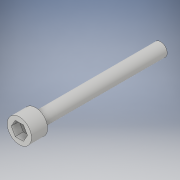
# Autodesk Inventor part: RobotArm Rivet2
Saved by Autodesk Inventor 2018 (Build 220112000, 112)
## iProperties
Created: 2018-01-20
Part Number: RobotArm Rivet2
Material: Generic
Document SubType Name: Modeling
Designer: lopez.xavier
Density: 1 g/cm^3
Appearance: Default
Author: lopez.xavier
Autodesk Inventor part; units mm, degrees
ref_plane "YZ Plane" through (0, 0, 0) normal (1, 0, 0) x (0, 1, 0)
ref_plane "XZ Plane" through (0, 0, 0) normal (0, 1, 0) x (-1, 0, 0)
ref_plane "XY Plane" through (0, 0, 0) normal (0, 0, 1) x (1, 0, 0)
sketch "Sketch1" plane through (0, 0, 0) normal (0, 0, 1) x (1, 0, 0)
  circle A0 centre (0, 0) radius 3.81
  dimension "d0" = 7.62
  constraints: 1 centre point, 1 coincident
  measures "d0" diameter of A0
extrude "Extrusion1" add sketch "Sketch1" along normal blind 5.08
sketch "Sketch2" plane through (0, 0, 5.08) normal (0, 0, 1) x (1, 0, 0)
  line L0 (1.2832, 2.2225) -> (2.5663, 0)
  line L1 (2.5663, 0) -> (1.2832, -2.2225)
  line L2 (1.2832, -2.2225) -> (-1.2832, -2.2225)
  line L3 (-1.2832, -2.2225) -> (-2.5663, 0)
  line L4 (-2.5663, 0) -> (-1.2832, 2.2225)
  line L5 (-1.2832, 2.2225) -> (1.2832, 2.2225)
  line L6 (0, 0) -> (0.4307, 0)
  dimension "d3" = 4.445
  constraints: 14 end point, 1 coincident, 1 horizontal, 1 parallel, 13 other
  measures "d3" distance between parallel lines of L2 L5
extrude "Extrusion2" cut sketch "Sketch2" against normal blind 2.54
sketch "Sketch3" plane through (0, 0, 0) normal (0, 0, -1) x (-1, 0, 0)
  circle A0 centre (0, 0) radius 2.0701
  dimension "d6" = 4.1402
  constraints: 1 centre point, 1 coincident
  measures "d6" diameter of A0
extrude "Extrusion3" add sketch "Sketch3" along normal blind 39.37
body "Solid1"
